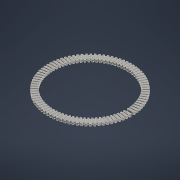
# Autodesk Inventor part: P028
Saved by Autodesk Inventor 2021.3 (Build 253353000, 353)
## iProperties
Company: HES-SO
Created: 2022-06-15
Part Number: P028
Material: Steel
Document SubType Name: Modeling
Designer: HER & ZAE
Density: 7.85 g/cm^3
Appearance: Steel
Mass: 1.08949 g
Surface Area: 7.71892 cm^2
Volume: 0.138789 cm^3
Author: HER & ZAE
Title: Segment racleur
Autodesk Inventor part; units mm, degrees
ref_plane "YZ Plane" through (0, 0, 0) normal (1, 0, 0) x (0, 1, 0)
ref_plane "XZ Plane" through (0, 0, 0) normal (0, 1, 0) x (-1, 0, 0)
ref_plane "XY Plane" through (0, 0, 0) normal (0, 0, 1) x (1, 0, 0)
sketch "Sketch2" plane through (0, 0, 0) normal (0, 0, 1) x (1, 0, 0)
  circle A0 centre (0, 0) radius 13 construction
  circle A1 centre (0, 0) radius 15 construction
  line L0 (-21, 0) -> (21, 0) construction
  line L1 (14.9977, 0) -> (14.9977, -0.1794) construction
  line L2 (14.9977, 0) -> (14.9977, -0.2618) construction
  line L3 (0, 0) -> (14.9977, 0.2618) construction
  line L4 (0, 0) -> (14.9977, -0.2618) construction
  line L5 (14.9977, 0.2618) -> (14.9977, 0) construction
  line L6 (12.998, 0.2269) -> (14.9977, 0.2618)
  line L7 (12.998, -0.2269) -> (14.9977, -0.2618)
  arc A2 (12.998, 0.2269) -> (12.998, -0.2269) centre (0, 0) ccw
  arc A3 (14.9977, 0.2618) -> (14.9977, -0.2618) centre (0, 0) ccw
  point P0 (14.9977, -0.2618)
  dimension "d1" = 2
  dimension "d2" = 2
  dimension "d14" = 30
  constraints: 14 end point, 8 point on circle, 4 centre point, 4 coincident, 4 collinear, 4 point on line, 2 vertical, 1 concentric, 1 perpendicular
  measures "d1" radial gap between concentric circles of A1 A0
  measures "d2" angle of L4 L3
  measures "d14" diameter of A1
extrude "Extrusion1" add sketch "Sketch2" along normal blind 0.4
sketch "Sketch3" plane through (0, 0, 0.4) normal (0, 0, 1) x (1, 0, 0)
  line L0 (12.998, 0.2269) -> (14.9977, 0.2618) construction
  arc A0 (14.9977, 0.2618) -> (14.9977, -0.2618) centre (0, 0) ccw construction
  line L1 (14.9977, -0.2618) -> (12.998, -0.2269) construction
  arc A1 (12.998, 0.2269) -> (12.998, -0.2269) centre (0, 0) ccw construction
  line L2 (0, 0) -> (14.9794, 0.785) construction
  arc A2 (14.9977, 0.2618) -> (14.9977, -0.2618) centre (0, 0) ccw construction
  arc A3 (12.998, 0.2269) -> (12.998, -0.2269) centre (0, 0) ccw projected
  line L3 (12.9822, 0.6804) -> (14.9794, 0.785)
  line L4 (12.998, 0.2269) -> (14.9977, 0.2618) projected
  line L5 (14.9977, 0.2618) -> (12.998, 0.2269)
  arc A4 (12.998, 0.2269) -> (12.9822, 0.6804) centre (0, 0) ccw
  arc A5 (14.9977, 0.2618) -> (14.9794, 0.785) centre (0, 0) ccw
  dimension "d5" = 2
  constraints: 6 end point, 6 point on circle, 2 centre point, 2 coincident, 2 collinear, 1 point on line
  measures "d5" angle of L2 L0
extrude "Extrusion2" add sketch "Sketch3" along normal blind 0.4
sketch "Sketch4" plane through (0, 0, 0) normal (0, 0, -1) x (-1, 0, 0)
  line L0 (-12.998, 0.2269) -> (-14.9977, 0.2618) construction
  arc A0 (-12.998, -0.2269) -> (-12.998, 0.2269) centre (0, 0) ccw construction
  line L1 (-14.9977, -0.2618) -> (-12.998, -0.2269) construction
  arc A1 (-14.9977, -0.2618) -> (-14.9977, 0.2618) centre (0, 0) ccw construction
  line L2 (-14.9794, 0.785) -> (-12.9822, 0.6804) construction
  arc A2 (-12.9822, 0.6804) -> (-12.998, 0.2269) centre (0, 0) ccw construction
  line L3 (-12.998, 0.2269) -> (-14.9977, 0.2618) construction
  arc A3 (-14.9794, 0.785) -> (-14.9977, 0.2618) centre (0, 0) ccw construction
  arc A4 (-14.9977, -0.2618) -> (-14.9977, 0.2618) centre (0, 0) ccw construction
  line L4 (0, 0) -> (-14.9429, 1.3073) construction
  line L5 (-12.9822, 0.6804) -> (-14.9794, 0.785)
  line L6 (-14.9429, 1.3073) -> (-12.9505, 1.133)
  arc A5 (-12.998, -0.2269) -> (-12.998, 0.2269) centre (0, 0) ccw projected
  line L7 (-14.9794, 0.785) -> (-12.9822, 0.6804) projected
  arc A6 (-12.9505, 1.133) -> (-12.9822, 0.6804) centre (0, 0) ccw
  arc A7 (-14.9429, 1.3073) -> (-14.9794, 0.785) centre (0, 0) ccw
  dimension "d8" = 2
  constraints: 6 end point, 6 point on circle, 2 centre point, 2 coincident, 1 collinear, 1 point on line
  measures "d8" angle of L4 L2
extrude "Extrusion3" add sketch "Sketch4" along normal blind 0.4
pattern_circular "Circular Pattern1" count 84 over 354 about axis through (0, 0, -10) along (0, 0, 1) of "Extrusion2", "Extrusion3"
body "Solid1"
